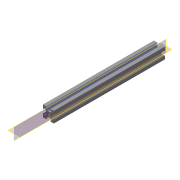
# Autodesk Inventor part: 00_VSlot_20mm_250mm
Saved by Autodesk Inventor 2019.4 (Build 234330000, 330)
## iProperties
Created: 2021-10-12
Part Number: 00_VSlot_20mm_250mm
Material: Generic
Document SubType Name: Modeling
Designer: diederichbenedict
Density: 1 g/cm^3
Appearance: Default
Author: diederichbenedict
Autodesk Inventor part; units mm, degrees
ref_plane "YZ Plane" through (0, 0, 0) normal (1, 0, 0) x (0, 1, 0)
ref_plane "XZ Plane" through (0, 0, 0) normal (0, 1, 0) x (-1, 0, 0)
ref_plane "XY Plane" through (0, 0, 0) normal (0, 0, 1) x (1, 0, 0)
sketch "Sketch1" plane through (0, 0, 0) normal (0, 0, 1) x (1, 0, 0)
  line L0 (1.7678, -1.7678) -> (3.9962, 0.4607) projected
  arc A0 (0, -2.5) -> (1.7678, -1.7678) centre (0, 0) ccw projected
  line L1 (-3.0076, -2.5) -> (0, -2.5) projected
  arc A1 (-4.7754, -1.7678) -> (-3.0076, -2.5) centre (-3.0076, 0) ccw projected
  line L2 (-7.0038, 0.4607) -> (-4.7754, -1.7678) projected
  line L3 (-7.0038, 2.4) -> (-7.0038, 0.4607) projected
  line L4 (-5.0038, 2.4) -> (-7.0038, 2.4) projected
  arc A2 (-5.0038, 2.4) -> (-4.6038, 2.8) centre (-5.0038, 2.8) ccw projected
  line L5 (-5.7038, 3.9) -> (-4.6038, 2.8) projected
  line L6 (-11.1038, 3.9) -> (-5.7038, 3.9) projected
  arc A3 (-11.1038, 3.9) -> (-11.5038, 3.5) centre (-11.1038, 3.5) ccw projected
  line L7 (-11.5038, -1.9) -> (-11.5038, 3.5) projected
  line L8 (-10.4038, -3) -> (-11.5038, -1.9) projected
  arc A4 (-10.4038, -3) -> (-10.0038, -2.6) centre (-10.4038, -2.6) ccw projected
  line L9 (-10.0038, -0.6) -> (-10.0038, -2.6) projected
  line L10 (-8.0645, -0.6) -> (-10.0038, -0.6) projected
  line L11 (-5.836, -2.8284) -> (-8.0645, -0.6) projected
  arc A5 (-5.1038, -4.5962) -> (-5.836, -2.8284) centre (-7.6038, -4.5962) ccw projected
  line L12 (-5.1038, -7.6038) -> (-5.1038, -4.5962) projected
  arc A6 (-5.836, -9.3716) -> (-5.1038, -7.6038) centre (-7.6038, -7.6038) ccw projected
  line L13 (-8.0645, -11.6) -> (-5.836, -9.3716) projected
  line L14 (-10.0038, -11.6) -> (-8.0645, -11.6) projected
  line L15 (-10.0038, -9.6) -> (-10.0038, -11.6) projected
  arc A7 (-10.0038, -9.6) -> (-10.4038, -9.2) centre (-10.4038, -9.6) ccw projected
  line L16 (-11.5038, -10.3) -> (-10.4038, -9.2) projected
  line L17 (-11.5038, -15.7) -> (-11.5038, -10.3) projected
  arc A8 (-11.5038, -15.7) -> (-11.1038, -16.1) centre (-11.1038, -15.7) ccw projected
  line L18 (-5.7038, -16.1) -> (-11.1038, -16.1) projected
  line L19 (-4.6038, -15) -> (-5.7038, -16.1) projected
  arc A9 (-4.6038, -15) -> (-5.0038, -14.6) centre (-5.0038, -15) ccw projected
  line L20 (-7.0038, -14.6) -> (-5.0038, -14.6) projected
  line L21 (-7.0038, -12.6607) -> (-7.0038, -14.6) projected
  line L22 (-4.7754, -10.4322) -> (-7.0038, -12.6607) projected
  arc A10 (-3.0076, -9.7) -> (-4.7754, -10.4322) centre (-3.0076, -12.2) ccw projected
  line L23 (0, -9.7) -> (-3.0076, -9.7) projected
  arc A11 (1.7678, -10.4322) -> (0, -9.7) centre (0, -12.2) ccw projected
  line L24 (3.9962, -12.6607) -> (1.7678, -10.4322) projected
  line L25 (3.9962, -14.6) -> (3.9962, -12.6607) projected
  line L26 (1.9962, -14.6) -> (3.9962, -14.6) projected
  arc A12 (1.9962, -14.6) -> (1.5962, -15) centre (1.9962, -15) ccw projected
  line L27 (2.6962, -16.1) -> (1.5962, -15) projected
  line L28 (8.0962, -16.1) -> (2.6962, -16.1) projected
  arc A13 (8.0962, -16.1) -> (8.4962, -15.7) centre (8.0962, -15.7) ccw projected
  line L29 (8.4962, -10.3) -> (8.4962, -15.7) projected
  line L30 (7.3962, -9.2) -> (8.4962, -10.3) projected
  arc A14 (7.3962, -9.2) -> (6.9962, -9.6) centre (7.3962, -9.6) ccw projected
  line L31 (6.9962, -11.6) -> (6.9962, -9.6) projected
  line L32 (5.0569, -11.6) -> (6.9962, -11.6) projected
  line L33 (2.8284, -9.3716) -> (5.0569, -11.6) projected
  arc A15 (2.0962, -7.6038) -> (2.8284, -9.3716) centre (4.5962, -7.6038) ccw projected
  line L34 (2.0962, -4.5962) -> (2.0962, -7.6038) projected
  arc A16 (2.8284, -2.8284) -> (2.0962, -4.5962) centre (4.5962, -4.5962) ccw projected
  line L35 (5.0569, -0.6) -> (2.8284, -2.8284) projected
  line L36 (6.9962, -0.6) -> (5.0569, -0.6) projected
  line L37 (6.9962, -2.6) -> (6.9962, -0.6) projected
  arc A17 (6.9962, -2.6) -> (7.3962, -3) centre (7.3962, -2.6) ccw projected
  line L38 (8.4962, -1.9) -> (7.3962, -3) projected
  line L39 (8.4962, 3.5) -> (8.4962, -1.9) projected
  arc A18 (8.4962, 3.5) -> (8.0962, 3.9) centre (8.0962, 3.5) ccw projected
  line L40 (2.6962, 3.9) -> (8.0962, 3.9) projected
  line L41 (1.5962, 2.8) -> (2.6962, 3.9) projected
  arc A19 (1.5962, 2.8) -> (1.9962, 2.4) centre (1.9962, 2.8) ccw projected
  line L42 (3.9962, 2.4) -> (1.9962, 2.4) projected
  line L43 (3.9962, 0.4607) -> (3.9962, 2.4) projected
  circle A20 centre (-1.5038, -6.1) radius 2.5 projected
  point P0 (0, 0)
extrude "Extrusion1" add sketch "Sketch1" along normal blind 250
ref_plane "Work Plane1" through (-1.5038, -15.7, 0) normal (-1, 0, 0) x (0, 0, 1)
ref_plane "Work Plane2" through (-11.1038, -6.1, 0) normal (0, 1, 0) x (1, 0, 0)
body "Solid1"
